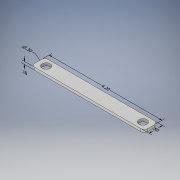
# Autodesk Inventor part: Side Rod V1
Saved by Autodesk Inventor 2018 (Build 220112000, 112)
## iProperties
Created: 2019-12-11
Part Number: Side Rod V1
Material: Generic
Document SubType Name: Modeling
Designer: AOFUser
Density: 1 g/cm^3
Appearance: Default
Author: AOFUser
Autodesk Inventor part; units mm, degrees
ref_plane "YZ Plane" through (0, 0, 0) normal (1, 0, 0) x (0, 1, 0)
ref_plane "XZ Plane" through (0, 0, 0) normal (0, 1, 0) x (-1, 0, 0)
ref_plane "XY Plane" through (0, 0, 0) normal (0, 0, 1) x (1, 0, 0)
sketch "Sketch1" plane through (0, 0, 0) normal (0, 1, 0) x (-1, 0, 0)
  line L0 (0, 0) -> (-106.68, 0)
  line L1 (-106.68, 0) -> (-106.68, -12.7)
  line L2 (-106.68, -12.7) -> (0, -12.7)
  line L3 (0, -12.7) -> (0, 0)
  dimension "d0" = 106.68
  dimension "d1" = 12.7
  constraints: 8 end point, 2 parallel, 1 horizontal, 1 perpendicular
  measures "d0" distance of L2.end L1.end
  measures "d1" distance of L1.end L0.end
extrude "Extrusion1" add sketch "Sketch1" along normal blind 2.54
fillet "Fillet1" radius 3.175 4 edges at (106.68, 1.27, 0) (106.68, 1.27, -12.7) (0, 1.27, 0) (0, 1.27, -12.7)
sketch "Sketch2" plane through (0, 2.54, 0) normal (0, 1, 0) x (1, 0, 0)
  line L0 (106.68, 3.175) -> (106.68, 9.525) projected
  line L1 (106.68, 6.35) -> (99.06, 6.35)
  line L2 (0, 6.35) -> (7.62, 6.35)
  circle A0 centre (99.06, 6.35) radius 3.81
  circle A1 centre (7.62, 6.35) radius 3.81
  point P0 (0, 0)
  dimension "d5" = 7.62
  dimension "d6" = 7.62
  dimension "d7" = 7.62
  dimension "d8" = 7.62
  constraints: 4 end point, 2 centre point, 2 coincident, 2 horizontal, 1 midpoint
  measures "d5" distance of L1.start L1.end
  measures "d6" distance of L2.start L2.end
  measures "d7" diameter of A0
  measures "d8" diameter of A1
extrude "Extrusion2" cut sketch "Sketch2" against normal blind 2.54 contours A0
sketch "Sketch3" plane through (0, 2.54, 0) normal (0, 1, 0) x (1, 0, 0)
  line L0 (0, 9.525) -> (0, 3.175) projected
  line L1 (0, 6.35) -> (7.62, 6.35)
  circle A0 centre (7.62, 6.35) radius 3.81
  point P0 (0, 0)
  dimension "d11" = 7.62
  dimension "d12" = 7.62
  constraints: 2 end point, 1 centre point, 1 coincident, 1 horizontal, 1 midpoint
  measures "d11" distance of L1.start L1.end
  measures "d12" diameter of A0
hole "Hole1" at (7.62, 2.54, -6.35) direction (0, -1, 0) diameter 7.62 end through all
body "Solid1"
